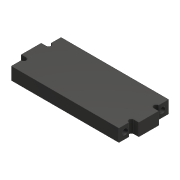
# Autodesk Inventor part: 頭_メインフレームセンター２
Saved by Autodesk Inventor 2017.3 (Build 213256000, 256)
## iProperties
Part Number: 頭_メインフレームセンター２
Material: アセタール樹脂、黒
Document SubType Name: Modeling
Designer: haya
Mass: 9.25538 g
Surface Area: 33.31 cm^2
Volume: 6.495 cm^3
Density: 1.425 g/cm^3
Appearance: 滑らか - 黒
Author: haya
Autodesk Inventor part; units mm, degrees
ref_plane "YZ Plane" through (0, 0, 0) normal (1, 0, 0) x (0, 1, 0)
ref_plane "XZ Plane" through (0, 0, 0) normal (0, 1, 0) x (-1, 0, 0)
ref_plane "XY Plane" through (0, 0, 0) normal (0, 0, 1) x (1, 0, 0)
sketch "スケッチ1" plane through (0, 0, 0) normal (0, 0, 1) x (1, 0, 0)
  line L0 (0, 0) -> (43.3, 0)
  line L1 (43.3, 20) -> (0, 20)
  line L2 (0, 10) -> (43.3, 10) construction
  line L3 (43.3, 14) -> (45.3, 14)
  line L4 (45.3, 14) -> (45.3, 6)
  line L5 (45.3, 6) -> (43.3, 6)
  arc A0 (43.3, 16) -> (43.3, 14) centre (43.3, 15) ccw
  arc A1 (43.3, 6) -> (43.3, 4) centre (43.3, 5) ccw
  line L6 (43.3, 0) -> (43.3, 4)
  line L7 (43.3, 16) -> (43.3, 20)
  line L8 (21.65, 20) -> (21.65, 0) construction
  line L9 (0, 14) -> (-2, 14)
  line L10 (-2, 14) -> (-2, 6)
  line L11 (-2, 6) -> (0, 6)
  arc A2 (0, 14) -> (0, 16) centre (0, 15) ccw
  arc A3 (0, 4) -> (0, 6) centre (0, 5) ccw
  line L12 (0, 0) -> (0, 4)
  line L13 (0, 16) -> (0, 20)
  dimension "d0" = 43.3
  dimension "d1" = 20
  dimension "d5" = 8
  dimension "d6" = 2
  constraints: 28 end point, 9 symmetric about line, 8 point on circle, 5 perpendicular, 4 centre point, 2 horizontal, 2 midpoint, 2 parallel, 2 point on line, 1 tangent, 5 other
  measures "d0" distance of L0.start L0.end
  measures "d1" distance of L1.end L0.start
  measures "d5" distance of L3.end L4.end
  measures "d6" diameter of A0
extrude "押し出し1" add sketch "スケッチ1" along normal blind 5
sketch "スケッチ3" plane through (43.3, 0, 0) normal (1, 0, 0) x (0, 0, -1)
  line L0 (0, 0) -> (-5, 0) projected
  line L1 (-2.5, 0) -> (-2.5, 20) construction
  line L2 (0, 20) -> (-5, 20) projected
  line L3 (-2.5, 10) -> (0, 10) construction
  line L4 (0, 6) -> (0, 14) projected
  point P0 (-2.5, 17.5)
  point P1 (-2.5, 2.5)
  dimension "d7" = 15
  constraints: 4 end point, 4 midpoint, 1 point on line, 1 symmetric about line
  measures "d7" distance of point (-2.5, 2.5) point (-2.5, 17.5)
hole "穴1" at (43.3, 17.5, 2.5) at (43.3, 2.5, 2.5) direction (-1, 0, 0) diameter 2.4 depth 8 tip angle 118
sketch "スケッチ4" plane through (0, 16, 0) normal (-1, 0, 0) x (0, 0, 1)
  circle A0 centre (2.5, 1.5) radius 1.2 projected
  circle A1 centre (2.5, -13.5) radius 1.2 projected
  circle A2 centre (2.5, -13.5) radius 1.2 projected
  point P0 (0, -16)
hole "穴2" at (0, 17.5, 2.5) at (0, 2.5, 2.5) direction (1, 0, 0) diameter 2.4 depth 8 tip angle 118
